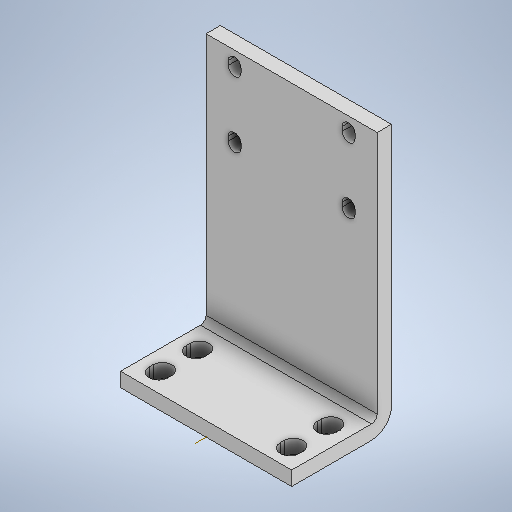
# Autodesk Inventor part: TS_V1_Fallmagazin_Haltewinkel_Fuehrung_int
Saved by Autodesk Inventor 2025.2 (Build 292293000, 293)
## iProperties
Created: 2025-06-16
Part Number: TS_V1_Fallmagazin_Haltewinkel_Fuehrung_int
Material: Generisch
Document SubType Name: Modeling
Designer: tino
Density: 1 g/cm^3
Appearance: Vorgabe
Author: tino
Autodesk Inventor part; units mm, degrees
ref_plane "YZ Plane" through (0, 0, 0) normal (1, 0, 0) x (0, 1, 0)
ref_plane "XZ Plane" through (0, 0, 0) normal (0, 1, 0) x (-1, 0, 0)
ref_plane "XY Plane" through (0, 0, 0) normal (0, 0, 1) x (1, 0, 0)
sketch "Skizze1" plane through (0, 0, 0) normal (1, 0, 0) x (0, 1, 0)
  line L0 (5, 92.5) -> (0, 92.5)
  line L1 (0, 92.5) -> (0, 0)
  line L2 (0, 0) -> (5, 0)
  line L3 (5, 0) -> (5, 92.5)
  line L4 (-37, 0) -> (12, 0) projected
  line L5 (0, 0) -> (-30, 0)
  line L6 (-30, 0) -> (-30, 5)
  line L7 (-30, 5) -> (0, 5)
  line L8 (0, 5) -> (0, 0)
  dimension "d0" = 5
  dimension "d1" = 92.5
  dimension "d3" = 5
  dimension "d4" = 35
  constraints: 16 end point, 4 parallel, 2 horizontal, 2 perpendicular, 1 collinear, 1 point on line
  measures "d0" distance of L2.end L1.end
  measures "d1" distance of L1.end L0.end
  measures "d3" distance of L5.end L6.end
  measures "d4" distance between parallel lines of L6 L3
extrude "Extrusion1" add sketch "Skizze1" along normal mid plane 60
fillet "Rundung1" radius 2 1 edges at (0, 0, 5)
fillet "Rundung2" radius 7 1 edges at (0, 5, 0)
sketch "Skizze2" plane through (-30, 0, 92.5) normal (0, -1, 0) x (1, 0, 0)
  line L0 (0, -92.5) -> (60, -92.5) projected
  line L1 (60, 0) -> (60, -85.5) projected
  line L2 (0, -85.5) -> (0, 0) projected
  line L3 (10, -2) -> (10, -2)
  line L4 (12.25, -4.25) -> (12.25, -5.75)
  line L5 (10, -8) -> (10, -8)
  line L6 (7.75, -5.75) -> (7.75, -4.25)
  line L7 (7.75, -2) -> (12.25, -8) construction
  line L8 (12.25, -2) -> (7.75, -8) construction
  arc A0 (10, -2) -> (7.75, -4.25) centre (10, -4.25) ccw
  arc A1 (12.25, -4.25) -> (10, -2) centre (10, -4.25) ccw
  arc A2 (7.75, -5.75) -> (10, -8) centre (10, -5.75) ccw
  arc A3 (10, -8) -> (12.25, -5.75) centre (10, -5.75) ccw
  point P0 (30, -92.5)
  point P1 (10, -5)
  point P2 (10, -2)
  point P3 (10, -8)
  dimension "d12" = 60
  dimension "d13" = 10
  dimension "d14" = 4.5
  dimension "d15" = 6
  dimension "d16" = 2.25
  dimension "d17" = 87.5
  constraints: 12 end point, 8 point on circle, 8 point on line, 8 tangent, 4 centre point, 3 equal radius, 2 midpoint, 2 parallel, 1 horizontal, 1 perpendicular
  measures "d12" distance between parallel lines of L1 L2
  measures "d13" distance from line of L2 point (10, -5)
  measures "d14" distance of L7.end L8.end
  measures "d15" distance of L8.start L7.end
  measures "d16" radius of A0
  measures "d17" distance from line of L0 point (10, -5)
extrude "Extrusion2" cut sketch "Skizze2" against normal blind 50
pattern_linear "Rechteckige Anordnung1" count 2 spacing 40 along (1, 0, 0) count 2 spacing 23 along (0, 0, -1) of "Extrusion2"
sketch "Skizze3" plane through (-30, -30, 5) normal (0, 0, 1) x (1, 0, 0)
  line L0 (7, 11) -> (7, 11)
  line L1 (10.3, 7.7) -> (10.3, 6.3)
  line L2 (7, 3) -> (7, 3)
  line L3 (3.7, 6.3) -> (3.7, 7.7)
  line L4 (3.7, 11) -> (10.3, 3) construction
  line L5 (10.3, 11) -> (3.7, 3) construction
  arc A0 (7, 11) -> (3.7, 7.7) centre (7, 7.7) ccw
  arc A1 (3.7, 6.3) -> (7, 3) centre (7, 6.3) ccw
  arc A2 (7, 3) -> (10.3, 6.3) centre (7, 6.3) ccw
  arc A3 (10.3, 7.7) -> (7, 11) centre (7, 7.7) ccw
  line L6 (0, 0) -> (0, 28) projected
  line L7 (0, 0) -> (60, 0) projected
  point P0 (30, 30)
  point P1 (7, 7)
  point P2 (7, 3)
  dimension "d26" = 6.6
  dimension "d27" = 8
  dimension "d28" = 3.3
  dimension "d29" = 7
  dimension "d30" = 7
  constraints: 12 end point, 8 point on circle, 8 point on line, 8 tangent, 4 centre point, 3 equal radius, 2 midpoint, 2 parallel, 1 horizontal, 1 perpendicular
  measures "d26" distance of L4.end L5.end
  measures "d27" distance of L5.start L4.end
  measures "d28" radius of A0
  measures "d29" distance from line of L6 point (7, 7)
  measures "d30" distance from line of L7 point (7, 7)
extrude "Extrusion3" cut sketch "Skizze3" against normal through all
pattern_linear "Rechteckige Anordnung2" count 2 spacing 46 along (1, 0, 0) count 2 spacing 13 along (0, 1, 0) of "Extrusion3"
